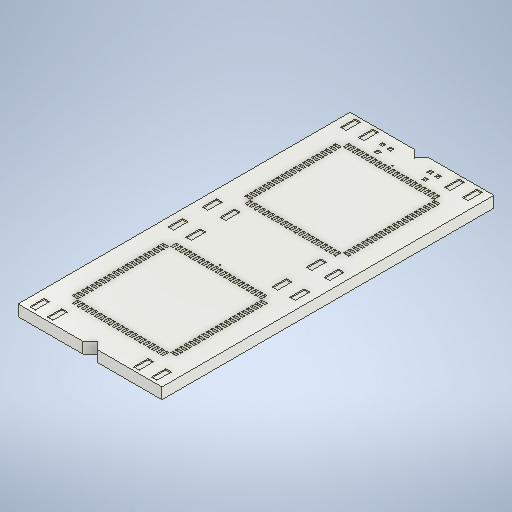
# Autodesk Inventor part: body
Saved by Autodesk Inventor 2025 (Build 290162000, 162)
## iProperties
Created: 2025-09-08
Part Number: body
Material: white ceramic
Document SubType Name: Modeling
Designer: jirne
Density: 1 g/cm^3
Appearance: Generic
Author: jirne
Autodesk Inventor part; units mm, degrees
sketch "Sketch1" plane through (0, 0, 0) normal (0, 0, 1) x (1, 0, 0)
  line L0 (0, 0) -> (0, 76.2)
  line L1 (0, 76.2) -> (14.8649, 76.2)
  line L2 (14.8649, 76.2) -> (16.51, 74.5549)
  line L3 (16.51, 74.5549) -> (18.1551, 76.2)
  line L4 (18.1551, 76.2) -> (33.02, 76.2)
  line L5 (33.02, 76.2) -> (33.02, 0)
  line L6 (33.02, 0) -> (18.1551, 0)
  line L7 (18.1551, 0) -> (16.51, 1.6451)
  line L8 (16.51, 1.6451) -> (14.8649, 0)
  line L9 (14.8649, 0) -> (0, 0)
  dimension "d0" = 76.2
  dimension "d1" = 33.02
  constraints: 20 end point, 7 equal length, 5 perpendicular, 2 point on line, 1 parallel, 1 vertical
  measures "d0" distance of L0.start L0.end
  measures "d1" distance of L4.end L0.end
extrude "Extrusion1" add sketch "Sketch1" along normal blind 2.54
sketch "Sketch2" plane through (0, 0, 2.54) normal (0, 0, 1) x (1, 0, 0)
  line L0 (6.096, 7.62) -> (6.604, 7.62)
  line L1 (6.604, 7.62) -> (6.604, 6.35)
  line L2 (6.604, 6.35) -> (6.096, 6.35)
  line L3 (6.096, 6.35) -> (6.096, 7.62)
  line L4 (0, 76.2) -> (0, 0) projected
  line L5 (0, 0) -> (14.8649, 0) projected
  point P0 (6.096, 6.35)
  dimension "d4" = 0.508
  dimension "d5" = 1.27
  dimension "d6" = 6.096
  dimension "d7" = 6.35
  constraints: 8 end point, 2 parallel, 1 horizontal, 1 perpendicular
  measures "d4" distance of L0.start L0.end
  measures "d5" distance of L2.end L0.start
  measures "d6" distance from line of L4 point (6.096, 6.35)
  measures "d7" distance from line of L5 point (6.096, 6.35)
extrude "Extrusion2" cut sketch "Sketch2" against normal blind 10
pattern_linear "Rectangular Pattern1" count 21 spacing 1.016 along (1, 0, 0) count 2 spacing 22.606 along (0, 1, 0) of "Extrusion2"
sketch "Sketch3" plane through (0, 0, 2.54) normal (0, 0, 1) x (1, 0, 0)
  line L0 (4.572, 8.382) -> (5.842, 8.382)
  line L1 (5.842, 8.382) -> (5.842, 7.874)
  line L2 (5.842, 7.874) -> (4.572, 7.874)
  line L3 (4.572, 7.874) -> (4.572, 8.382)
  line L4 (6.096, 7.62) -> (6.604, 7.62) projected
  line L5 (6.096, 6.35) -> (6.096, 7.62) projected
  point P0 (0, 0)
  point P1 (6.096, 6.985)
  dimension "d16" = 1.27
  dimension "d17" = 0.508
  dimension "d18" = 0.254
  dimension "d19" = 0.254
  constraints: 8 end point, 2 parallel, 1 horizontal, 1 midpoint, 1 perpendicular
  measures "d16" distance of L0.start L0.end
  measures "d17" distance of L2.end L0.start
  measures "d18" distance from line of L4 point (5.842, 7.874)
  measures "d19" horizontal distance of point (6.096, 6.985) point (5.842, 7.874)
extrude "Extrusion3" cut sketch "Sketch3" against normal blind 10
pattern_linear "Rectangular Pattern2" count 21 spacing 1.016 along (0, 1, 0) count 2 spacing 22.606 along (1, 0, 0) of "Extrusion3"
ref_plane "Work Plane1" through (0, 38.1, 0) normal (0, -1, 0) x (1, 0, 0)
mirror "Mirror1" about plane through (0, 38.1, 0) normal (0, -1, 0) of "Extrusion3", "Rectangular Pattern2", "Extrusion2", "Rectangular Pattern1"
sketch "Sketch4" plane through (0, 0, 2.54) normal (0, 0, 1) x (1, 0, 0)
  line L0 (1.905, 0.762) -> (3.175, 0.762)
  line L1 (3.175, 0.762) -> (3.175, 4.064)
  line L2 (3.175, 4.064) -> (1.905, 4.064)
  line L3 (1.905, 4.064) -> (1.905, 0.762)
  line L4 (5.969, 0.762) -> (7.239, 0.762)
  line L5 (7.239, 0.762) -> (7.239, 4.064)
  line L6 (7.239, 4.064) -> (5.969, 4.064)
  line L7 (5.969, 4.064) -> (5.969, 0.762)
  line L8 (0, 0) -> (14.8649, 0) projected
  line L9 (0, 76.2) -> (0, 0) projected
  point P0 (1.905, 0.762)
  point P1 (5.969, 0.762)
  dimension "d28" = 3.302
  dimension "d29" = 1.27
  dimension "d30" = 3.302
  dimension "d31" = 1.27
  dimension "d32" = 0.762
  dimension "d33" = 1.905
  dimension "d34" = 4.064
  constraints: 16 end point, 4 parallel, 2 horizontal, 2 perpendicular
  measures "d28" distance of L2.end L0.start
  measures "d29" distance of L1.end L2.end
  measures "d30" distance of L6.end L4.start
  measures "d31" distance of L5.end L6.end
  measures "d32" distance from line of L8 point (1.905, 0.762)
  measures "d33" distance from line of L9 point (1.905, 0.762)
  measures "d34" distance of point (1.905, 0.762) point (5.969, 0.762)
extrude "Extrusion4" cut sketch "Sketch4" against normal blind 0.254
pattern_linear "Rectangular Pattern3" count 2 spacing 23.876 along (1, 0, 0) count 2 spacing 31.75 along (0, 1, 0) of "Extrusion4"
mirror "Mirror2" about plane through (0, 38.1, 0) normal (0, -1, 0) of "Extrusion4", "Rectangular Pattern3"
ref_plane "Work Plane2" through (0, 0, 1.27) normal (0, 0, 1) x (1, 0, 0)
mirror "Mirror3" about plane through (0, 0, 1.27) normal (0, 0, 1) of "Extrusion4", "Rectangular Pattern3", "Mirror2"
sketch "Sketch5" plane through (0, 0, 2.54) normal (0, 0, 1) x (1, 0, 0)
  line L0 (10.668, 71.882) -> (11.43, 71.882)
  line L1 (11.43, 71.882) -> (11.43, 71.12)
  line L2 (11.43, 71.12) -> (10.668, 71.12)
  line L3 (10.668, 71.12) -> (10.668, 71.882)
  line L4 (9.779, 73.914) -> (10.541, 73.914)
  line L5 (10.541, 73.914) -> (10.541, 73.152)
  line L6 (10.541, 73.152) -> (9.779, 73.152)
  line L7 (9.779, 73.152) -> (9.779, 73.914)
  line L8 (11.557, 73.914) -> (12.319, 73.914)
  line L9 (12.319, 73.914) -> (12.319, 73.152)
  line L10 (12.319, 73.152) -> (11.557, 73.152)
  line L11 (11.557, 73.152) -> (11.557, 73.914)
  line L12 (14.8649, 76.2) -> (0, 76.2) projected
  line L13 (7.239, 75.438) -> (7.239, 72.136) projected
  point P0 (0, 0)
  point P1 (9.779, 71.12)
  point P2 (9.779, 71.12)
  dimension "d43" = 0.762
  dimension "d44" = 2.032
  dimension "d45" = 2.54
  dimension "d46" = 0.889
  dimension "d47" = 5.08
  dimension "d48" = 2.54
  constraints: 24 end point, 6 parallel, 5 equal length, 3 horizontal, 3 perpendicular, 1 collinear
  measures "d43" distance of L0.start L0.end
  measures "d44" distance of point (9.779, 71.12) point (9.779, 73.152)
  measures "d45" distance of L8.end L4.start
  measures "d46" distance of point (9.779, 71.12) point (10.668, 71.12)
  measures "d47" distance from line of L12 point (9.779, 71.12)
  measures "d48" distance from line of L13 point (9.779, 71.12)
extrude "Extrusion5" cut sketch "Sketch5" against normal blind 0.254
ref_plane "Work Plane3" through (16.51, 0, 0) normal (-1, 0, 0) x (0, 0, 1)
mirror "Mirror4" about plane through (16.51, 0, 0) normal (-1, 0, 0) of "Extrusion5"
sketch "Sketch6" plane through (0, 0, 2.54) normal (0, 0, 1) x (1, 0, 0)
  line L0 (15.24, 30.226) -> (15.748, 30.226) projected
  line L1 (15.24, 69.85) -> (15.748, 69.85) projected
  circle A0 centre (15.494, 70.485) radius 0.127
  circle A1 centre (15.494, 30.861) radius 0.127
  point P0 (0, 0)
  dimension "d51" = 0.635
  dimension "d52" = 0.635
  dimension "d53" = 0.254
  dimension "d54" = 0.254
  constraints: 2 centre point, 2 coincident
  measures "d51" distance from line of point (15.494, 30.861) L0
  measures "d52" distance from line of point (15.494, 70.485) L1
  measures "d53" diameter of A0
  measures "d54" diameter of A1
extrude "Extrusion6" cut sketch "Sketch6" against normal blind 0.254
body "Solid1"
